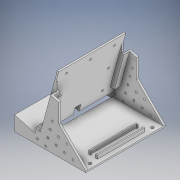
# Autodesk Inventor part: IPC Modular Stand
Saved by Autodesk Inventor 2022 (Build 260153000, 153)
## iProperties
Created: 2022-01-07
Part Number: IPC Modular Stand
Material: Generic
Document SubType Name: Modeling
Designer: solor
Density: 1 g/cm^3
Appearance: Default
Author: solor
Autodesk Inventor part; units mm, degrees
ref_plane "YZ Plane" through (0, 0, 0) normal (1, 0, 0) x (0, 1, 0)
ref_plane "XZ Plane" through (0, 0, 0) normal (0, 1, 0) x (-1, 0, 0)
sketch "Sketch1" plane through (0, 0, 0) normal (0, 0, 1) x (1, 0, 0)
  line L0 (0, 0) -> (0, -25.4)
  line L1 (124.1505, -25.4) -> (0, -25.4)
  line L2 (0, 0) -> (36.019, -9.6513)
  line L3 (36.019, -9.6513) -> (63.4797, 92.8335)
  line L4 (63.4797, 92.8335) -> (65.9331, 92.1761)
  line L5 (66.9992, 91.8904) -> (66.9734, 91.7938) construction
  line L6 (66.9992, 91.8904) -> (67.0992, 91.8904) construction
  line L7 (66.9734, 91.7938) -> (63.1692, 92.8131) construction
  line L8 (38.4724, -10.3087) -> (41.3489, 1.5865) construction
  line L9 (124.1505, -25.4) -> (124.1505, -22.86)
  line L10 (77.385, 24.1017) -> (124.1505, -22.86)
  circle A0 centre (59.4346, 56.2852) radius 1.7
  line L11 (59.4346, 56.2852) -> (55.5524, 41.7963) construction
  circle A1 centre (55.5524, 41.7963) radius 1.7
  line L12 (55.5524, 41.7963) -> (51.6701, 27.3074) construction
  circle A2 centre (51.6701, 27.3074) radius 1.7
  line L13 (51.6701, 27.3074) -> (47.7878, 12.8185) construction
  circle A3 centre (47.7878, 12.8185) radius 1.7
  line L14 (47.7878, 12.8185) -> (43.9055, -1.6704) construction
  circle A4 centre (43.9055, -1.6704) radius 1.7
  line L15 (43.9055, -1.6704) -> (40.0232, -16.1593) construction
  circle A5 centre (40.0232, -16.1593) radius 1.7
  line L16 (40.0232, -16.1593) -> (54.5121, -20.0416) construction
  line L17 (43.9055, -1.6704) -> (58.3944, -5.5527) construction
  line L18 (47.7878, 12.8185) -> (62.2767, 8.9362) construction
  line L19 (51.6701, 27.3074) -> (66.159, 23.4251) construction
  line L20 (62.2767, 8.9362) -> (76.7656, 5.0539) construction
  line L21 (76.7656, 5.0539) -> (91.2544, 1.1717) construction
  line L22 (58.3944, -5.5527) -> (72.8833, -9.4349) construction
  line L23 (72.8833, -9.4349) -> (87.3722, -13.3172) construction
  line L24 (87.3722, -13.3172) -> (101.861, -17.1995) construction
  circle A6 centre (66.159, 23.4251) radius 1.7
  circle A7 centre (62.2767, 8.9362) radius 1.7
  circle A8 centre (76.7656, 5.0539) radius 1.7
  circle A9 centre (91.2544, 1.1717) radius 1.7
  circle A10 centre (58.3944, -5.5527) radius 1.7
  circle A11 centre (72.8833, -9.4349) radius 1.7
  circle A12 centre (87.3722, -13.3172) radius 1.7
  circle A13 centre (101.861, -17.1995) radius 1.7
  circle A14 centre (54.5121, -20.0416) radius 1.7
  line L25 (55.5524, 41.7963) -> (70.0412, 37.914) construction
  line L26 (55.5524, 41.7963) -> (70.0412, 37.914) construction
  line L27 (59.4346, 56.2852) -> (73.9235, 52.4029) construction
  circle A15 centre (73.9235, 52.4029) radius 1.7
  circle A16 centre (70.0412, 37.914) radius 1.7
  line L28 (63.4797, 83.0197) -> (93.4515, 83.0197) construction
  line L29 (77.385, 24.1017) -> (77.385, 57.2859)
  line L30 (65.9331, 92.1761) -> (61.2291, 74.6204)
  line L31 (77.385, 57.2859) -> (61.2291, 61.6149)
  line L32 (77.385, 57.2859) -> (97.4769, 57.2859) construction
  line L33 (61.2291, 61.6149) -> (61.2291, 74.6204)
  line L34 (61.2291, 61.6149) -> (74.2346, 61.6149) construction
  point P0 (62.7398, 80.2585)
  point P1 (52.2165, 40.9849)
  dimension "d4" = 25.4
  dimension "d8" = 2.54
  dimension "d11" = 0.1
  dimension "d12" = 105
  dimension "d16" = 2.54
  dimension "d20" = 15
  dimension "d21" = 3.4
  dimension "d22" = 15
  dimension "d23" = 3.4
  dimension "d24" = 15
  dimension "d25" = 3.4
  dimension "d26" = 15
  dimension "d27" = 3.4
  dimension "d28" = 15
  dimension "d29" = 3.4
  dimension "d30" = 15
  dimension "d32" = 15
  dimension "d33" = 15
  dimension "d34" = 15
  dimension "d35" = 15
  dimension "d36" = 15
  dimension "d37" = 15
  dimension "d38" = 15
  dimension "d39" = 15
  dimension "d40" = 3.4
  dimension "d41" = 3.4
  dimension "d42" = 3.4
  dimension "d43" = 3.4
  dimension "d44" = 3.4
  dimension "d45" = 3.4
  dimension "d46" = 3.4
  dimension "d47" = 3.4
  dimension "d48" = 3.4
  dimension "d98" = 3.4
  dimension "d99" = 3.4
  dimension "d101" = 165
  dimension "d102" = 90
  constraints: 70 end point, 17 centre point, 17 coincident, 5 horizontal, 4 perpendicular, 2 equal length, 2 vertical, 1 point on line
  measures "d4" distance of L0.start L0.end
  measures "d8" distance of L3.end L4.end
  measures "d11" distance of L5.start L5.end
  measures "d12" angle of L5 L6
  measures "d16" distance of L1.start L9.end
  measures "d20" distance of L11.start L11.end
  measures "d21" diameter of A1
  measures "d22" distance of L12.start L12.end
  measures "d23" diameter of A2
  measures "d24" distance of L13.start L13.end
  measures "d25" diameter of A3
  measures "d26" distance of L14.start L14.end
  measures "d27" diameter of A4
  measures "d28" distance of L15.start L15.end
  measures "d29" diameter of A5
  measures "d30" distance of L16.start L16.end
  measures "d32" distance of L17.start L17.end
  measures "d33" distance of L18.start L18.end
  measures "d34" distance of L19.start L19.end
  measures "d35" distance of L20.start L20.end
  measures "d36" distance of L21.start L21.end
  measures "d37" distance of L22.start L22.end
  measures "d38" distance of L23.start L23.end
  measures "d39" distance of L24.start L24.end
  measures "d40" diameter of A6
  measures "d41" diameter of A7
  measures "d42" diameter of A8
  measures "d43" diameter of A9
  measures "d44" diameter of A10
  measures "d45" diameter of A11
  measures "d46" diameter of A12
  measures "d47" diameter of A13
  measures "d48" diameter of A14
  measures "d98" diameter of A15
  measures "d99" diameter of A16
  measures "d101" angle of L32 L31
  measures "d102" angle of L34 L33
extrude "Extrusion1" add sketch "Sketch1" along normal blind 138.85 contours L2 L3 L4 L30 L33 L31 L29 L10 L9 L1 L0 | A15 | A16
ref_plane "Work Plane1" through (0, 0, 69.425) normal (0, 0, 1) x (1, 0, 0)
sketch "Sketch3" plane through (0, 0, 69.425) normal (0, 0, 1) x (1, 0, 0)
  line L0 (63.4797, 92.8335) -> (36.019, -9.6513) construction
  line L1 (36.019, -9.6513) -> (35.2425, -12.549) construction
  line L2 (0, 0) -> (0, -25.4) construction
  line L3 (0, -25.4) -> (124.1505, -25.4) construction
  line L4 (124.1505, -25.4) -> (124.1505, -22.86) construction
  line L5 (124.1505, -22.86) -> (77.385, 24.1017) construction
  line L6 (65.9331, 92.1761) -> (63.4797, 92.8335) construction
  line L7 (63.4797, 92.8335) -> (36.019, -9.6513) construction
  line L8 (36.019, -9.6513) -> (0, 0) construction
  circle A0 centre (40.0232, -16.1593) radius 1.7 construction
  circle A1 centre (54.5121, -20.0416) radius 1.7 construction
  circle A2 centre (101.861, -17.1995) radius 1.7 construction
  circle A3 centre (87.3722, -13.3172) radius 1.7 construction
  circle A4 centre (72.8833, -9.4349) radius 1.7 construction
  circle A5 centre (58.3944, -5.5527) radius 1.7 construction
  circle A6 centre (91.2544, 1.1717) radius 1.7 construction
  circle A7 centre (76.7656, 5.0539) radius 1.7 construction
  circle A8 centre (62.2767, 8.9362) radius 1.7 construction
  circle A9 centre (66.159, 23.4251) radius 1.7 construction
  circle A10 centre (43.9055, -1.6704) radius 1.7 construction
  circle A11 centre (47.7878, 12.8185) radius 1.7 construction
  circle A12 centre (51.6701, 27.3074) radius 1.7 construction
  circle A13 centre (55.5524, 41.7963) radius 1.7 construction
  circle A14 centre (59.4346, 56.2852) radius 1.7 construction
  line L9 (35.2425, -12.549) -> (0, -3.1058)
  line L10 (0, -3.1058) -> (0, -25.4)
  line L11 (0, -25.4) -> (35.2425, -25.4)
  line L12 (35.2425, -25.4) -> (35.2425, -22.86)
  line L13 (35.2425, -22.86) -> (124.1505, -22.86)
  line L14 (108.7659, -7.4108) -> (106.9661, -9.2031) construction
  line L15 (35.2425, -12.549) -> (37.6959, -13.2064)
  line L16 (37.6959, -13.2064) -> (63.4797, 83.0197)
  line L17 (63.4797, 83.0197) -> (124.1505, -22.86)
  line L18 (77.385, 57.2859) -> (61.2291, 61.6149) projected
  line L19 (61.2291, 61.6149) -> (61.2291, 74.6204) projected
  line L20 (61.2291, 74.6204) -> (65.9331, 92.1761) projected
  line L21 (77.385, 24.1017) -> (77.385, 57.2859) projected
  dimension "d53" = 3
  dimension "d54" = 2.54
  constraints: 20 end point, 3 point on line, 2 perpendicular, 1 collinear
  measures "d53" distance of L0.end L1.end
  measures "d54" distance of L11.end L12.end
extrude "Extrusion2" cut sketch "Sketch3" along normal mid plane 131.85
sketch "Sketch4" plane through (0, 0, 138.85) normal (0.258819, 0.9659258, 0) x (0.9659258, -0.258819, 0)
  line L0 (-42.009, 64.425) -> (74.0386, 64.425)
  line L1 (74.0386, 64.425) -> (74.0386, 74.425)
  line L2 (74.0386, 74.425) -> (-42.009, 74.425)
  line L3 (-42.009, 74.425) -> (-42.009, 64.425)
  line L4 (-42.009, 64.425) -> (74.0386, 74.425) construction
  line L5 (74.0386, 64.425) -> (-42.009, 74.425) construction
  point P0 (0, 138.85)
  point P1 (16.0148, 69.425)
  dimension "d58" = 10
  constraints: 12 end point, 2 midpoint, 2 parallel, 1 horizontal, 1 perpendicular
  measures "d58" distance of L1.end L0.end
extrude "Extrusion3" cut sketch "Sketch4" along normal blind 10 and the other way blind 3
sketch "Sketch6" plane through (63.4797, 92.8335, 0) normal (-0.9659258, 0.258819, 0) x (0, 0, 1)
  line L0 (0, 0) -> (138.85, 0) projected
  line L1 (69.425, 0) -> (69.425, -12.238)
  line L2 (69.425, -12.238) -> (27.683, -12.238)
  line L3 (69.425, -12.238) -> (111.167, -12.238)
  line L4 (27.683, 0) -> (27.683, -52.897) construction
  line L5 (27.683, 0) -> (27.683, -93.762) construction
  circle A0 centre (27.683, -12.238) radius 1.775
  circle A1 centre (27.683, -52.897) radius 1.775
  circle A2 centre (27.683, -93.762) radius 1.775
  circle A3 centre (69.425, -12.238) radius 1.775
  circle A4 centre (111.167, -12.238) radius 1.775
  circle A5 centre (111.167, -52.897) radius 1.775
  circle A6 centre (111.167, -93.762) radius 1.775
  point P0 (0, -106.1)
  dimension "d84" = 12.238
  dimension "d85" = 41.742
  dimension "d86" = 41.742
  dimension "d89" = 52.897
  dimension "d90" = 93.762
  dimension "d91" = 3.55
  constraints: 12 coincident, 10 end point, 7 centre point, 2 horizontal, 2 vertical, 1 midpoint, 1 perpendicular, 1 point on line
  measures "d84" distance of L1.start L1.end
  measures "d85" distance of L1.end L2.end
  measures "d86" distance of L1.end L3.end
  measures "d89" distance of L4.start L4.end
  measures "d90" distance of L4.start L5.end
  measures "d91" diameter of A0
sketch "Sketch7" plane through (35.2425, -22.86, 3.5) normal (0, 1, 0) x (1, 0, 0)
  line L0 (67.6836, -105.355) -> (79.1836, -105.355)
  line L1 (79.1836, -105.355) -> (79.1836, -26.495)
  line L2 (79.1836, -26.495) -> (67.6836, -26.495)
  line L3 (67.6836, -26.495) -> (67.6836, -105.355)
  line L4 (67.6836, -105.355) -> (79.1836, -26.495) construction
  line L5 (79.1836, -105.355) -> (67.6836, -26.495) construction
  line L6 (65.6836, -107.355) -> (81.1836, -107.355)
  line L7 (81.1836, -107.355) -> (81.1836, -24.495)
  line L8 (81.1836, -24.495) -> (65.6836, -24.495)
  line L9 (65.6836, -24.495) -> (65.6836, -107.355)
  point P0 (-35.2425, 3.5)
  point P1 (73.4336, -65.925)
  dimension "d74" = 11.5
  dimension "d75" = 78.86
  dimension "d76" = 2
  constraints: 20 end point, 4 parallel, 2 midpoint, 2 perpendicular, 1 horizontal, 3 other
  measures "d74" distance of L2.end L1.end
  measures "d75" distance of L1.end L0.end
  measures "d76" distance between parallel lines of L3 L9
extrude "Extrusion5" add sketch "Sketch7" along normal blind 6
sketch "Sketch8" plane through (35.2425, -16.86, 3.5) normal (0, 1, 0) x (1, 0, 0)
  line L0 (67.6836, -26.495) -> (79.1836, -26.495) projected
  line L1 (79.1836, -26.495) -> (79.1836, -105.355) projected
  line L2 (69.4313, -110.9088) -> (77.4358, -110.9088)
  line L3 (77.4358, -110.9088) -> (77.4358, -20.9412)
  line L4 (77.4358, -20.9412) -> (69.4313, -20.9412)
  line L5 (69.4313, -20.9412) -> (69.4313, -110.9088)
  line L6 (69.4313, -110.9088) -> (77.4358, -20.9412) construction
  line L7 (77.4358, -110.9088) -> (69.4313, -20.9412) construction
  point P0 (-35.2425, 3.5)
  point P1 (73.4336, -26.495)
  point P2 (79.1836, -65.925)
  point P3 (73.4336, -65.925)
  constraints: 12 end point, 4 midpoint, 2 parallel, 1 horizontal, 1 perpendicular
extrude "Extrusion6" cut sketch "Sketch8" against normal blind 6
chamfer "Chamfer1" distance 1 angle 45 4 edges at (104.6738, -16.86, 109.855) (112.6783, -16.86, 109.855) (104.6738, -16.86, 28.995) (112.6783, -16.86, 28.995)
extrude "Extrusion7" cut sketch "Sketch6" against normal blind 8.4045
sketch "Sketch9" plane through (35.2425, -22.86, 3.5) normal (0, 1, 0) x (1, 0, 0)
  line L0 (81.1836, -107.355) -> (81.1836, -24.495) projected
  line L1 (64.2789, -11.5924) -> (81.1836, -11.5924)
  line L2 (81.1836, -11.5924) -> (81.1836, -120.2576)
  line L3 (81.1836, -120.2576) -> (64.2789, -120.2576)
  line L4 (64.2789, -120.2576) -> (64.2789, -11.5924)
  line L5 (64.2789, -11.5924) -> (81.1836, -120.2576) construction
  line L6 (81.1836, -11.5924) -> (64.2789, -120.2576) construction
  circle A0 centre (81.1836, -11.5924) radius 2.5
  circle A1 centre (81.1836, -120.2576) radius 2.5
  point P0 (-35.2425, 3.5)
  point P1 (72.7312, -65.925)
  dimension "d94" = 5
  constraints: 12 end point, 2 centre point, 2 coincident, 2 midpoint, 2 parallel, 1 horizontal, 1 perpendicular, 1 point on line
  measures "d94" diameter of A0
extrude "Extrusion8" cut sketch "Sketch9" against normal blind 8.4045 contours A1 L3 L2 | L2 L3 A1 | A0 L1 L2 | L2 L1 A0
extrude "Extrusion9" cut sketch "Sketch1" along normal blind 10 contours A15 | A16
sketch "Sketch10" plane through (0, 0, 0) normal (0, 0, -1) x (-1, 0, 0)
  line L0 (-36.019, -9.6513) -> (0, 0) projected
  line L1 (-62.7672, 61.2027) -> (-47.0564, 2.5692)
  line L2 (-62.7672, 61.2027) -> (-2.0653, 61.2027) construction
  line L3 (-47.0564, 2.5692) -> (-39.2934, 2.5692)
  line L4 (-48.9998, 0.008) -> (-65.2207, 60.5453)
  line L5 (-48.9998, 0.008) -> (-38.6071, 0.008)
  line L6 (-38.6071, 0.008) -> (-39.2934, 2.5692)
  line L7 (-65.2207, 60.5453) -> (-62.7672, 61.2027)
  line L8 (-62.7672, 61.2027) -> (-71.2427, 92.8335)
  line L9 (-71.2427, 92.8335) -> (-58.3017, 96.301)
  line L10 (-58.3017, 96.301) -> (-39.2934, 2.5692)
  line L11 (-77.385, 57.2859) -> (-61.2291, 61.6149) projected
  line L12 (-62.7672, 61.2027) -> (-61.2291, 61.6149)
  line L13 (-61.2291, 61.6149) -> (-61.2291, 74.6204) projected
  line L14 (-61.2291, 61.6149) -> (-61.2291, 74.6204)
  line L15 (-61.2291, 74.6204) -> (-41.923, 2.5692)
  point P0 (-65.9331, 92.1761)
  point P1 (-65.9331, 92.1761)
  dimension "d111" = 75
  dimension "d112" = 2.54
  constraints: 26 end point, 3 horizontal, 2 collinear, 2 perpendicular, 1 equal length, 1 point on line
  measures "d111" angle of L1 L2
  measures "d112" distance between parallel lines of L1 L4
extrude "Extrusion11" cut sketch "Sketch10" against normal blind 11 contours L11 L13 L15 L3 L1 | L8 L9 L10 L3 L15 L13 L11
extrude "Extrusion12" add sketch "Sketch10" against normal blind 13.54 contours L1 L3 L6 L5 L4 L7
sketch "Sketch11" plane through (0, 0, 138.85) normal (0, 0, 1) x (1, 0, 0)
  line L0 (71.2427, 92.8335) -> (58.3017, 96.301) projected
  line L1 (58.3017, 96.301) -> (39.2934, 2.5692) projected
  line L2 (38.6071, 0.008) -> (39.2934, 2.5692) projected
  line L3 (47.0564, 2.5692) -> (39.2934, 2.5692) projected
  line L4 (62.7672, 61.2027) -> (47.0564, 2.5692) projected
  line L5 (62.7672, 61.2027) -> (71.2427, 92.8335) projected
  line L6 (65.2207, 60.5453) -> (62.7672, 61.2027) projected
  line L7 (48.9998, 0.008) -> (65.2207, 60.5453) projected
  line L8 (39.2934, 2.5692) -> (47.0564, 2.5692) projected
  line L9 (48.9998, 0.008) -> (38.6071, 0.008) projected
  point P0 (0, 0)
extrude "Extrusion13" cut sketch "Sketch11" against normal blind 11 contours L5 L4 L3 L1 L0
extrude "Extrusion14" add sketch "Sketch11" against normal blind 13.54 contours L6 L7 L9 L2 L3 L4
sketch "Sketch12" plane through (0, 0, 13.54) normal (0, 0, 1) x (1, 0, 0)
  line L0 (61.2291, 61.6149) -> (61.2291, 74.6204) projected
  line L1 (61.2291, 74.6204) -> (41.923, 2.5692) projected
  line L2 (77.385, 57.2859) -> (61.2291, 61.6149) projected
  line L3 (62.7672, 61.2027) -> (47.0564, 2.5692) projected
  line L4 (39.2934, 2.5692) -> (47.0564, 2.5692) projected
  line L5 (62.7672, 61.2027) -> (47.0564, 2.5692) projected
  line L6 (47.0564, 2.5692) -> (39.2934, 2.5692) projected
  point P0 (0, 0)
extrude "Extrusion15" add sketch "Sketch12" against normal blind 2.54
sketch "Sketch13" plane through (0, 0, 125.31) normal (0, 0, -1) x (-1, 0, 0)
  line L0 (-61.2291, 74.6204) -> (-41.923, 2.5692) projected
  line L1 (-39.2934, 2.5692) -> (-47.0564, 2.5692) projected
  line L2 (-63.4797, 92.8335) -> (-39.2934, 2.5692) projected
  line L3 (-65.9331, 92.1761) -> (-63.4797, 92.8335) projected
  line L4 (-61.2291, 74.6204) -> (-65.9331, 92.1761) projected
  line L5 (-61.2291, 74.6204) -> (-61.2291, 61.6149) projected
  line L6 (-61.2291, 61.6149) -> (-62.7672, 61.2027) projected
  line L7 (-47.0564, 2.5692) -> (-62.7672, 61.2027) projected
  point P0 (0, 0)
extrude "Extrusion16" add sketch "Sketch13" against normal blind 2.54 contours L0 L1 L7 L6 L5
body "Solid1"
